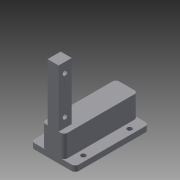
# Autodesk Inventor part: Autonomous - Encoder Mount
Saved by Autodesk Inventor 2014 (Build 180170000, 170)
## iProperties
Created: 2015-05-07
Part Number: Autonomous - Encoder Mount
Material: Generic
Document SubType Name: Modeling
Designer: WillHuie
Density: 1 g/cm^3
Appearance: Default
Author: WillHuie
Autodesk Inventor part; units mm, degrees
ref_plane "YZ Plane" through (0, 0, 0) normal (1, 0, 0) x (0, 1, 0)
ref_plane "XZ Plane" through (0, 0, 0) normal (0, 1, 0) x (-1, 0, 0)
ref_plane "XY Plane" through (0, 0, 0) normal (0, 0, 1) x (1, 0, 0)
sketch "Sketch1" plane through (0, 0, 0) normal (0, 1, 0) x (-1, 0, 0)
  line L0 (0, 0) -> (40.64, 0)
  line L1 (40.64, 0) -> (40.64, 67.945)
  line L2 (40.64, 67.945) -> (0, 67.945)
  line L3 (0, 67.945) -> (0, 0)
  line L4 (10.16, 0) -> (10.16, 67.945)
  line L5 (30.48, 0) -> (30.48, 67.945)
  dimension "d0" = 40.64
  dimension "d1" = 67.945
  constraints: 12 end point, 4 point on line, 3 parallel, 2 perpendicular, 1 horizontal
  measures "d0" distance of L0.start L0.end
  measures "d1" distance of L0.end L1.end
extrude "Extrusion1" add sketch "Sketch1" along normal blind 5.08
sketch "Sketch2" plane through (0, 5.08, 0) normal (0, 1, 0) x (1, 0, 0)
  line L0 (0, 0) -> (-40.64, 0) projected
  line L1 (-40.64, -67.945) -> (0, -67.945) projected
  line L2 (0, -67.945) -> (0, 0) projected
  line L3 (-10.16, 0) -> (-10.16, -67.945)
  line L4 (-30.48, 0) -> (-30.48, -67.945)
  constraints: 4 end point, 4 point on line, 1 parallel, 1 perpendicular
extrude "Extrusion2" add sketch "Sketch2" along normal blind 20.32 contours L3 L1 L4 L0
sketch "Sketch3" plane through (0, 25.4, 0) normal (0, 1, 0) x (1, 0, 0)
  line L0 (-30.48, -67.945) -> (-10.16, -67.945) projected
  line L1 (-10.16, -67.945) -> (-10.16, 0) projected
  line L2 (-25.4, -55.88) -> (-15.24, -55.88)
  line L3 (-25.4, -55.88) -> (-25.4, -67.945)
  line L4 (-15.24, -55.88) -> (-15.24, -67.945)
  point P0 (0, 0)
  constraints: 6 end point, 3 perpendicular, 2 point on line
extrude "Extrusion3" add sketch "Sketch3" along normal blind 52.705
sketch "Sketch4" plane through (-15.24, 25.4, 67.945) normal (1, 0, 0) x (0, 0, -1)
  circle A0 centre (6.0325, 8.89) radius 2.2225
  circle A1 centre (6.0325, 43.815) radius 2.2225
  point P0 (67.945, -25.4)
  dimension "d8" = 4.445
  dimension "d10" = 4.445
  constraints: 2 centre point
  measures "d8" diameter of A0
  measures "d10" diameter of A1
extrude "Extrusion4" cut sketch "Sketch4" against normal blind 52.705
sketch "Sketch5" plane through (0, 5.08, 0) normal (0, 1, 0) x (1, 0, 0)
  circle A0 centre (-5.08, -12.7) radius 2.2225
  circle A1 centre (-5.08, -55.245) radius 2.2225
  dimension "d14" = 4.445
  dimension "d16" = 4.445
  constraints: 2 centre point
  measures "d14" diameter of A0
  measures "d16" diameter of A1
extrude "Extrusion5" cut sketch "Sketch5" against normal blind 52.705
sketch "Sketch6" plane through (0, 5.08, 0) normal (0, 1, 0) x (1, 0, 0)
  circle A0 centre (-35.56, -12.7) radius 2.2225
  circle A1 centre (-35.56, -55.245) radius 2.2225
  point P0 (0, 0)
  dimension "d21" = 4.445
  dimension "d22" = 4.445
  constraints: 2 centre point
  measures "d21" diameter of A0
  measures "d22" diameter of A1
extrude "Extrusion6" cut sketch "Sketch6" against normal blind 52.705
fillet "Fillet1" radius 3.175 1 edges at (-40.64, 2.54, 0)
fillet "Fillet2" radius 3.175 1 edges at (-40.64, 2.54, 67.945)
fillet "Fillet3" radius 3.175 1 edges at (0, 2.54, 0)
fillet "Fillet4" radius 3.175 1 edges at (0, 2.54, 67.945)
fillet "Fillet7" radius 3.175 1 edges at (-10.16, 15.24, 67.945)
fillet "Fillet8" radius 3.175 1 edges at (-30.48, 15.24, 67.945)
fillet "Fillet9" radius 3.175 1 edges at (-10.16, 15.24, 0)
fillet "Fillet10" radius 3.175 1 edges at (-30.48, 15.24, 0)
body "Solid1"
